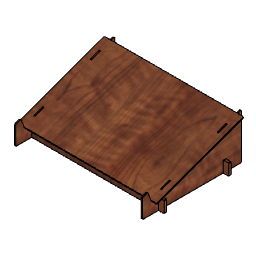
laptop_stand v2 (Autodesk Fusion 360 design; units mm, degrees)
Autodesk Fusion 360 part; units mm, degrees
sketch "Sketch1" plane through (0, 0, 0) normal (1, 0, 0) x (0, 1, 0) in component "Leg"
  line L0 (0, 0) -> (260, 0)
  line L1 (260, 0) -> (260, 120)
  line L2 (260, 120) -> (21.9167, 33.3447)
  line L3 (21.9167, 33.3447) -> (14, 55.0956)
  line L4 (14, 55.0956) -> (0, 50)
  line L5 (0, 50) -> (0, 0)
  dimension "d1" = 50
  dimension "d2" = 260
  dimension "d3" = 120
  dimension "d5" = 20
  dimension "d6" = 14
  dimension "d11" = 0
  dimension "d12" = 0
  dimension "d13" = 0
  dimension "d14" = 0
  dimension "d15" = 0
  dimension "d16" = 0
  dimension "d17" = 0
  dimension "d18" = 0
  constraint coincident L0.start L5.end
  constraint horizontal L0
  constraint perpendicular L0 L1
  constraint perpendicular L2 L3
  constraint perpendicular L0 L5
  constraint perpendicular L3 L4
  measures "d1" distance of L4.end L0.start
  measures "d2" distance of L0.start L0.end
  measures "d3" distance of L0.end L1.end
  measures "d5" angle of L0 L2
  measures "d6" horizontal distance of L3.end L4.end
extrude "Extrude1" add sketch "Sketch1" along normal blind 3 makes body 1 in component "Leg"
sketch "Sketch1 (2)" plane through (0, -8.153, 22.4003) normal (0, -0.34202, 0.939693) x (1, 0, 0) in component "Top"
  line L0 (0, 285.3625) -> (0, 31.9995)
  line L1 (0, 31.9995) -> (3, 31.9995)
  line L2 (3, 31.9995) -> (3, 285.3625)
  line L3 (3, 285.3625) -> (0, 285.3625)
  line L4 (-333, 285.3625) -> (-333, 31.9995)
  line L5 (-333, 31.9995) -> (-330, 31.9995)
  line L6 (-330, 31.9995) -> (-330, 285.3625)
  line L7 (-330, 285.3625) -> (-333, 285.3625)
  line L8 (-348, 275.3625) -> (18, 275.3625)
  line L9 (18, 275.3625) -> (18, 31.9995)
  line L10 (18, 31.9995) -> (-348, 31.9995)
  line L11 (-348, 31.9995) -> (-348, 275.3625)
  line L12 (0, 245.3625) -> (3, 245.3625)
  line L13 (3, 245.3625) -> (3, 220.3625)
  line L14 (3, 220.3625) -> (0, 220.3625)
  line L15 (0, 220.3625) -> (0, 245.3625)
  line L16 (-165, 275.3625) -> (-165, 31.9995) construction
  line L17 (-348, 153.681) -> (18, 153.681) construction
  line L18 (-330, 245.3625) -> (-333, 245.3625)
  line L19 (-330, 220.3625) -> (-330, 245.3625)
  line L20 (-333, 245.3625) -> (-333, 220.3625)
  line L21 (-333, 220.3625) -> (-330, 220.3625)
  line L22 (-330, 61.9995) -> (-333, 61.9995)
  line L23 (-333, 86.9995) -> (-330, 86.9995)
  line L24 (-330, 86.9995) -> (-330, 61.9995)
  line L25 (-333, 61.9995) -> (-333, 86.9995)
  line L26 (0, 61.9995) -> (3, 61.9995)
  line L27 (0, 86.9995) -> (0, 61.9995)
  line L28 (3, 61.9995) -> (3, 86.9995)
  line L29 (3, 86.9995) -> (0, 86.9995)
  dimension "d31" = 10
  dimension "d32" = 15
  dimension "d33" = 15
  dimension "d34" = 25
  dimension "d35" = 30
  constraint horizontal L8
  constraint vertical L9
  constraint horizontal L10
  constraint vertical L11
  constraint collinear L5 L10
  constraint horizontal L12
  constraint vertical L13
  constraint horizontal L14
  constraint vertical L15
  constraint coincident L2 L13.end
  constraint coincident L0 L12.start
  constraint midpoint L8 L16.start
  constraint midpoint L10 L16.end
  constraint midpoint L11 L17.start
  constraint midpoint L9 L17.end
  constraint symmetric L12.start L16 L18.start
  constraint symmetric L12.end L16 L18.end
  constraint symmetric L13.end L16 L20.end
  constraint symmetric L14.end L16 L19.start
  constraint symmetric L12.start L17 L26.start
  constraint symmetric L12.end L17 L26.end
  constraint symmetric L13.end L17 L28.end
  constraint symmetric L14.end L17 L27.start
  constraint symmetric L17 L18.start L22.start
  constraint symmetric L17 L18.end L22.end
  constraint symmetric L17 L20.end L23.start
  constraint symmetric L17 L19.start L23.end
  measures "d31" distance of L2.end L8
  measures "d32" distance of L2 L9
  measures "d33" distance of L4 L11
  measures "d34" distance of L12.end L13.end
  measures "d35" distance of L8 L12.end
extrude "Extrude1'" add sketch "Sketch1 (2)" against normal blind 3 separate body contours L0 L6 L8 L10 L15 L19 L24 L27 | L0 L2 L8 L12 | L0 L2 L14 L29 | L2 L8 L9 L10 L13 L28 | L4 L6 L8 L18 | L0 L1 L2 L10 L26 | L4 L8 L10 L11 L20 L25 | L4 L6 L21 L23 | L4 L5 L6 L10 L22 makes body 2 in component "Top"
combine "Combine1" operation cut target body 1 tool bodies 2 keep tools in component "Leg"
ref_plane "WorkPlane1" through (1.5, 215, 60) normal (0, 1, 0) x (0, 0, 1) in component "Support"
sketch "Sketch1 (3)" plane through (1.5, 215, 60) normal (0, 1, 0) x (1, 0, 0) in component "Support"
  line L0 (-1.5, 60) -> (-1.5, -60)
  line L1 (-1.5, -60) -> (1.5, -60)
  line L2 (1.5, -60) -> (1.5, 60)
  line L3 (1.5, 60) -> (-1.5, 60)
  line L4 (-334.5, 60) -> (-334.5, -60)
  line L5 (-334.5, -60) -> (-331.5, -60)
  line L6 (-331.5, -60) -> (-331.5, 60)
  line L7 (-331.5, 60) -> (-334.5, 60)
  line L8 (16.5, 30) -> (-349.5, 30)
  line L9 (-349.5, 30) -> (-349.5, 60)
  line L10 (-349.5, 60) -> (16.5, 60)
  line L11 (16.5, 60) -> (16.5, 30)
  line L12 (-349.5, 29.4743) -> (-349.5, -53.7607)
  line L13 (16.5, -53.7607) -> (16.5, 29.4743)
  line L14 (16.5, 45) -> (-349.5, 45)
  dimension "d39" = 30
  constraint horizontal L8
  constraint vertical L9
  constraint horizontal L10
  constraint vertical L11
  constraint collinear L9 L12
  constraint collinear L11 L13
  constraint collinear L3 L10
  constraint midpoint L11 L14.start
  constraint midpoint L9 L14.end
  measures "d39" distance of L8.start L10.end
extrude "Extrude1''" add sketch "Sketch1 (3)" along normal mid plane 6 separate body contours L0 L2 L3 L10 L14 | L0 L6 L10 L14 | L0 L6 L8 L14 | L2 L10 L11 L14 | L4 L6 L7 L10 L14 | L2 L8 L11 L14 | L4 L9 L10 L14 | L4 L8 L9 L14 makes body 3 in component "Support"
ref_plane "WorkPlane2" through (1.5, 130, 60) normal (0, 1, 0) x (0, 0, 1) in component "Support"
fillet "Fillet1" radius 1 8 edges at (3, 215, 30) (0, 215, 30) (18, 215, 30) (18, 215, 0) (-330, 215, 30) (-333, 215, 30) (-348, 215, 30) (-348, 215, 0) on bodies 3 in component "Support"
mirror "Mirror1" about plane through (1.5, 130, 60) normal (0, 1, 0) of bodies 3 makes body 4 in component "Support"
fillet "Fillet1'" radius 2 10 edges at (1.5, 260, 120) (1.5, 250.6031, 116.5798) (1.5, 222.4123, 106.3192) (1.5, 198.92, 97.7687) (1.5, 73.5998, 52.1559) (1.5, 50.1074, 43.6054) (1.5, 14, 55.0956) (1.5, 0, 50) (1.5, 0, 0) (1.5, 260, 0) on bodies 1 in component "Leg"
fillet "Fillet1''" radius 2 4 edges at (18, 22.4297, 31.9352) (18, 251.1161, 115.1703) (-348, 22.4297, 31.9352) (-348, 251.1161, 115.1703) on bodies 2 in component "Top"
combine "Combine2" operation cut target body 1 tool bodies 3 4 keep tools in component "Leg"
component "Leg" placed x (1, 0, 0) y (0, 1, 0) z (0, 0, 1) at (-333, 0, 0)
component "Leg" placed x (1, 0, 0) y (0, 1, 0) z (0, 0, 1) at (0, 0, 0)
component "Top" placed x (1, 0, 0) y (0, 1, 0) z (0, 0, 1) at (0, 0, 0)
component "Support" placed x (1, 0, 0) y (0, 1, 0) z (0, 0, 1) at (0, 0, 0)
equation "legwidth = 3 mm"
equation "legdistance = 330 mm"
equation "d9 = legwidth"
equation "d22 = legdistance"
equation "d36 = -legwidth"
equation "d40 = legwidth"
